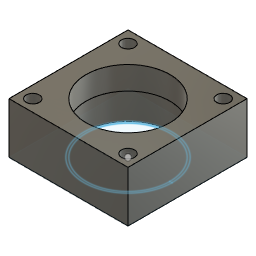
BearingBlock v7 (Autodesk Fusion 360 archive; units mm, degrees)
design "BearingBlock" references "tormach 770mx"
Autodesk Fusion 360 part; units mm, degrees
sketch "Sketch1" plane through (0, 0, 0) normal (0, 1, 0) x (1, 0, 0)
  line L0 (0, 0) -> (30, 0)
  line L1 (30, 0) -> (30, -30)
  line L2 (30, -30) -> (0, -30)
  line L3 (0, -30) -> (0, 0)
  dimension "d1" = 30
  constraint horizontal L0
  constraint vertical L1
  constraint horizontal L2
  constraint vertical L3
  constraint coincident L0.start L3.end
  measures "d1" distance of L0.start L0.end
extrude "Extrude1" add sketch "Sketch1" along normal blind 12.8
sketch "Sketch2" plane through (0, 12.8, 0) normal (0, 1, 0) x (-1, 0, 0)
  line L0 (0, 30) -> (-30, 30)
  line L1 (-30, 30) -> (-30, 0)
  line L2 (-30, 0) -> (0, 0)
  line L3 (0, 0) -> (0, 30)
  line L4 (0, 15) -> (-30, 15) construction
  line L5 (-15, 0) -> (-15, 30) construction
  circle A0 centre (-15, 15) radius 4.5
  line L6 (-3, 27) -> (-27, 27) construction
  line L7 (-27, 27) -> (-27, 3) construction
  line L8 (-27, 3) -> (-3, 3) construction
  line L9 (-3, 3) -> (-3, 27) construction
  line L10 (-3, 27) -> (-27, 3) construction
  line L11 (-27, 27) -> (-3, 3) construction
  point P0 (-15, 15)
  point P1 (-15, 15)
  point P2 (-27, 3)
  point P3 (-3, 3)
  point P4 (-3, 27)
  point P5 (-27, 27)
  dimension "d7" = 9
  dimension "d14" = 24
  dimension "d15" = 24
  constraint midpoint L3 L4.start
  constraint midpoint L1 L4.end
  constraint midpoint L2 L5.start
  constraint midpoint L0 L5.end
  constraint midpoint L4 P1
  constraint coincident P1 P0
  constraint horizontal L6
  constraint perpendicular L6 L7
  constraint parallel L6 L8
  constraint parallel L7 L9
  constraint coincident L10 P1
  constraint coincident L11 P1
  constraint coincident P2 L7.end
  constraint coincident P3 L8.end
  constraint coincident P4 L6.start
  constraint coincident P5 L6.end
  measures "d7" diameter of A0
  measures "d14" distance of P2 P3
  measures "d15" distance of P5 P2
sketch "Sketch3" plane through (0, 0, 0) normal (0, -1, 0) x (1, 0, 0)
  line L0 (30, 30) -> (0, 30)
  line L1 (0, 30) -> (0, 0)
  line L2 (0, 0) -> (30, 0)
  line L3 (30, 0) -> (30, 30)
  circle A0 centre (15, 15) radius 11.075
  circle A1 centre (15, 15) radius 10.55
  dimension "d11" = 22.15
  dimension "d31" = 21.1
  constraint concentric A0 A1
  measures "d11" diameter of A0
  measures "d31" diameter of A1
hole "Hole2" at (3, 12.8, 3) direction (0, -1, 0) diameter 3.3 end through all
hole "Hole3" at (27, 12.8, 3) direction (0, -1, 0) diameter 3.3 end through all
hole "Hole4" at (27, 12.8, 27) direction (0, -1, 0) diameter 3.3 end through all
hole "Hole5" at (3, 12.8, 27) direction (0, -1, 0) diameter 3.3 end through all
extrude "Extrude7" cut sketch "Sketch3" against normal blind 7 contours A0
extrude "Extrude8" cut sketch "Sketch3" against normal through all contours A1
